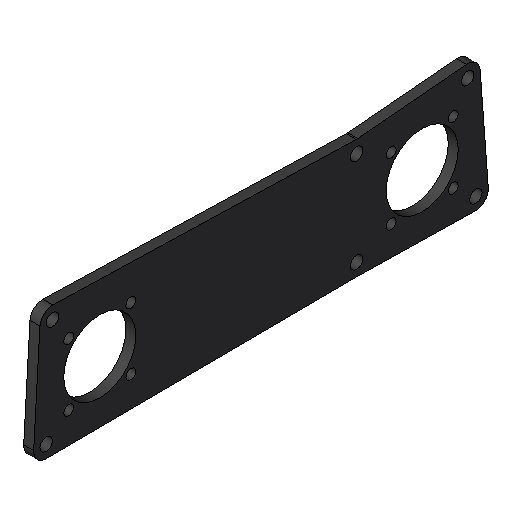
# Autodesk Inventor part: ChassiMotorMount3.3
Saved by Autodesk Inventor 2023 (Build 270158000, 158)
## iProperties
Created: 2022-09-16
Part Number: ChassiMotorMount3.3
Material: Generic
Document SubType Name: Modeling
Designer: deli
Density: 1 g/cm^3
Appearance: Default
Author: deli
Autodesk Inventor part; units mm, degrees
ref_plane "YZ Plane" through (0, 0, 0) normal (1, 0, 0) x (0, 1, 0)
ref_plane "XZ Plane" through (0, 0, 0) normal (0, 1, 0) x (-1, 0, 0)
ref_plane "XY Plane" through (0, 0, 0) normal (0, 0, 1) x (1, 0, 0)
sketch "Sketch1" plane through (0, 0, 0) normal (1, 0, 0) x (0, 1, 0)
  circle A0 centre (39.3404, 43.2624) radius 2
  circle A1 centre (5.9097, 45.2669) radius 2
  circle A2 centre (6.6549, -53.7618) radius 2
  circle A3 centre (5.9097, -91.791) radius 2
  circle A4 centre (39.8287, -89.1951) radius 2
  arc A5 (43.3389, 43.152) -> (39.5798, 47.2552) centre (39.3404, 43.2624) ccw
  circle A6 centre (36.6644, -53.7618) radius 4 construction
  arc A7 (40.134, -93.1835) -> (43.8126, -88.8357) centre (39.8287, -89.1951) ccw
  arc A8 (1.9104, -91.7126) -> (6.2149, -95.7793) centre (5.9097, -91.791) ccw
  arc A9 (2.6557, -53.6834) -> (2.6557, -53.6834) centre (6.6549, -53.7618) ccw
  arc A10 (6.1491, 49.2597) -> (1.9098, 45.2367) centre (5.9097, 45.2669) ccw
  line L0 (1.9098, 45.2367) -> (2.6557, -53.6834)
  line L1 (2.6557, -53.6834) -> (1.9104, -91.7126)
  line L2 (39.5798, 47.2552) -> (6.1491, 49.2597)
  line L3 (40.134, -93.1835) -> (6.2149, -95.7793)
  arc A11 (40.6659, -53.6514) -> (40.6806, -54.1212) centre (44.6644, -53.7618) ccw
  line L4 (43.3389, 43.152) -> (40.6659, -53.6514)
  line L5 (43.8126, -88.8357) -> (40.6806, -54.1212)
  line L6 (6.6549, -53.7618) -> (44.6644, -53.7618) construction
  circle A12 centre (21.6597, 28.1642) radius 11.5
  circle A13 centre (21.6597, -74.6883) radius 11.5
  circle A14 centre (31.5592, 38.0637) radius 1.6
  circle A15 centre (31.5592, 18.2647) radius 1.6
  circle A16 centre (11.7602, 18.2647) radius 1.6
  circle A17 centre (11.7602, 38.0637) radius 1.6
  circle A18 centre (11.7602, -64.7888) radius 1.6
  circle A19 centre (31.5592, -64.7888) radius 1.6
  circle A20 centre (31.5592, -84.5878) radius 1.6
  circle A21 centre (11.7602, -84.5878) radius 1.6
  line L7 (31.5592, 38.0637) -> (31.5592, 18.2647) construction
  line L8 (31.5592, 18.2647) -> (11.7602, 18.2647) construction
  line L9 (11.7602, 18.2647) -> (11.7602, 38.0637) construction
  line L10 (11.7602, 38.0637) -> (31.5592, 38.0637) construction
  line L11 (31.5592, 38.0637) -> (11.7602, 18.2647) construction
  line L12 (11.7602, 38.0637) -> (31.5592, 18.2647) construction
  line L13 (31.5592, -64.7888) -> (31.5592, -84.5878) construction
  line L14 (31.5592, -84.5878) -> (11.7602, -84.5878) construction
  line L15 (11.7602, -84.5878) -> (11.7602, -64.7888) construction
  line L16 (11.7602, -64.7888) -> (31.5592, -64.7888) construction
  line L17 (11.7602, -84.5878) -> (31.5592, -64.7888) construction
  line L18 (11.7602, -64.7888) -> (31.5592, -84.5878) construction
  circle A22 centre (36.6644, -53.7618) radius 2
  circle A23 centre (5.9097, 45.2669) radius 2 projected
  circle A24 centre (39.3404, 43.2624) radius 2 projected
  circle A25 centre (21.6597, 28.1642) radius 7 projected
  circle A26 centre (21.6597, -74.6883) radius 7 projected
  circle A27 centre (5.9097, -91.791) radius 2 projected
  circle A28 centre (39.8287, -89.1951) radius 2 projected
  circle A29 centre (36.6644, -53.7618) radius 2 projected
  circle A30 centre (6.6549, -53.7618) radius 2 projected
  point P0 (0, 0)
  point P1 (45.7953, -76.7779)
  point P2 (49.3122, -19.5779)
  point P3 (21.0827, -58.3908)
  point P4 (19.3835, -56.016)
  point P5 (17.555, -42.4349)
  point P6 (17.3497, -15.1829)
  point P7 (53.615, -21.1734)
  point P8 (53.7299, -25.9433)
  point P9 (21.0179, -9.8497)
  point P10 (19.0255, -12.7465)
  dimension "d0" = 8
  dimension "d1" = 8
  dimension "d2" = 8
  dimension "d3" = 8
  dimension "d4" = 8
  dimension "d5" = 8
  dimension "d6" = 8
  dimension "d8" = 23
  dimension "d9" = 23
  dimension "d12" = 3.2
  dimension "d13" = 3.2
  dimension "d14" = 3.2
  dimension "d15" = 3.2
  dimension "d16" = 3.2
  dimension "d17" = 3.2
  dimension "d18" = 3.2
  dimension "d19" = 3.2
  dimension "d20" = 28
  dimension "d23" = 28
  dimension "d24" = 4
  constraints: 38 end point, 23 centre point, 12 point on circle, 12 tangent, 9 concentric, 6 coincident, 6 perpendicular, 5 equal radius, 4 midpoint, 4 vertical, 2 point on line, 1 horizontal
  measures "d0" diameter of A5
  measures "d1" diameter of A10
  measures "d2" diameter of A9
  measures "d3" diameter of A6
  measures "d4" diameter of A7
  measures "d5" diameter of A8
  measures "d6" diameter of A11
  measures "d8" diameter of A12
  measures "d9" diameter of A13
  measures "d12" diameter of A14
  measures "d13" diameter of A15
  measures "d14" diameter of A16
  measures "d15" diameter of A17
  measures "d16" diameter of A18
  measures "d17" diameter of A19
  measures "d18" diameter of A20
  measures "d19" diameter of A21
  measures "d20" distance of L7.start L8.end
  measures "d23" distance of L14.end L13.start
  measures "d24" diameter of A0
extrude "Extrusion1" add sketch "Sketch1" along normal blind 3.175 contours A9 | L4 A11 L5 A7 L3 A8 L1 L0 A10 L2 A5
equation "\"d1\" = d0"
equation "\"d2\" = d0"
equation "\"d3\" = d0"
equation "\"d4\" = d0"
equation "\"d5\" = d0"
equation "\"d6\" = d0"
equation "\"d9\" = d8"
equation "\"d13\" = d12"
equation "\"d14\" = d12"
equation "\"d15\" = d12"
equation "\"d16\" = d12"
equation "\"d17\" = d12"
equation "\"d18\" = d12"
equation "\"d19\" = d12"
equation "\"d23\" = d20"
body "Solid1"
